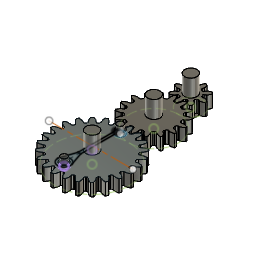
SqueezeFan v3 (Autodesk Fusion 360 design; units mm, degrees)
description: Spur Gear; Diametrial Pitch: 8.000000; Num Teeth: 24; Pressure Angle: 20.000000; Backlash: 0.00 in
description: Spur Gear; Diametrial Pitch: 8.000000; Num Teeth: 16; Pressure Angle: 20.000000; Backlash: 0.05 in
description: Spur Gear; Diametrial Pitch: 8.000000; Num Teeth: 8; Pressure Angle: 20.000000; Backlash: 0.00 in
Autodesk Fusion 360 part; units mm, degrees
(part 1 of 11)
sketch "Sketch1" plane through (0, 0, 0) normal (0, 0, 1) x (1, 0, 0) in component "Spur Gear (24 teeth)"
  circle A0 centre (0, 0) radius 34.2392
  circle A1 centre (0, 0) radius 6.35
extrude "Extrude1" add sketch "Sketch1" along normal blind 12.7 makes body 1 in component "Spur Gear (24 teeth)"
sketch "Sketch2" plane through (0, 0, 0) normal (0, 0, 1) x (1, 0, 0) in component "Spur Gear (24 teeth)"
  spline S0 degree 5 poles (35.6868, -2.8738) (35.7028, -2.8751) (35.735, -2.8772) (35.7832, -2.8793) (35.8475, -2.8797) (35.9281, -2.8771) (36.0087, -2.8722) (36.0893, -2.8659) (36.17, -2.8589) (36.2507, -2.8513) (36.3314, -2.8432) (36.4121, -2.8344) (36.4928, -2.8246) (36.5735, -2.8138) (36.6542, -2.8018) (36.7349, -2.7889) (36.8156, -2.775) (36.8963, -2.7604) (36.9769, -2.7452) (37.0576, -2.7294) (37.1382, -2.713) (37.2187, -2.696) (37.2993, -2.6783) (37.3798, -2.6599) (37.4603, -2.6409) (37.5408, -2.6212) (37.6212, -2.6008) (37.7016, -2.5799) (37.7819, -2.5584) (37.8622, -2.5364) (37.9425, -2.5139) (38.0227, -2.4907) (38.1029, -2.4671) (38.183, -2.4429) (38.2631, -2.4181) (38.3431, -2.3929) (38.4231, -2.3671) (38.503, -2.3408) (38.5829, -2.314) (38.6627, -2.2867) (38.7425, -2.2589) (38.8222, -2.2307) (38.9018, -2.2019) (38.9814, -2.1727) (39.061, -2.143) (39.1404, -2.1129) (39.2198, -2.0822) (39.2992, -2.0512) (39.3785, -2.0196) (39.4577, -1.9876) (39.5369, -1.9552) (39.6159, -1.9224) (39.695, -1.889) (39.7739, -1.8553) (39.8528, -1.8211) (39.9316, -1.7865) (40.0103, -1.7515) (40.089, -1.7161) (40.1676, -1.6802) (40.2461, -1.644) (40.3245, -1.6073) (40.4029, -1.5702) (40.4811, -1.5327) (40.5593, -1.4948) (40.6374, -1.4565) (40.7155, -1.4178) (40.7934, -1.3787) (40.8713, -1.3392) (40.9491, -1.2993) (41.0268, -1.259) (41.1044, -1.2184) (41.1664, -1.1855) (41.2129, -1.1607) (41.2439, -1.1441) (41.2594, -1.1358) knots 0 0 0 0 0 0 0.01428571 0.02857143 0.04285714 0.05714286 0.07142857 0.08571429 0.1 0.11428571 0.12857143 0.14285714 0.15714286 0.17142857 0.18571429 0.2 0.21428571 0.22857143 0.24285714 0.25714286 0.27142857 0.28571429 0.3 0.31428571 0.32857143 0.34285714 0.35714286 0.37142857 0.38571429 0.4 0.41428571 0.42857143 0.44285714 0.45714286 0.47142857 0.48571429 0.5 0.51428571 0.52857143 0.54285714 0.55714286 0.57142857 0.58571429 0.6 0.61428571 0.62857143 0.64285714 0.65714286 0.67142857 0.68571429 0.7 0.71428571 0.72857143 0.74285714 0.75714286 0.77142857 0.78571429 0.8 0.81428571 0.82857143 0.84285714 0.85714286 0.87142857 0.88571429 0.9 0.91428571 0.92857143 0.94285714 0.95714286 0.97142857 0.98571429 1 1 1 1 1 1
  spline S1 degree 5 poles (35.6868, 2.8738) (35.7028, 2.8751) (35.735, 2.8772) (35.7832, 2.8793) (35.8475, 2.8797) (35.9281, 2.8771) (36.0087, 2.8722) (36.0893, 2.8659) (36.17, 2.8589) (36.2507, 2.8513) (36.3314, 2.8432) (36.4121, 2.8344) (36.4928, 2.8246) (36.5735, 2.8138) (36.6542, 2.8018) (36.7349, 2.7889) (36.8156, 2.775) (36.8963, 2.7604) (36.9769, 2.7452) (37.0576, 2.7294) (37.1382, 2.713) (37.2187, 2.696) (37.2993, 2.6783) (37.3798, 2.6599) (37.4603, 2.6409) (37.5408, 2.6212) (37.6212, 2.6008) (37.7016, 2.5799) (37.7819, 2.5584) (37.8622, 2.5364) (37.9425, 2.5139) (38.0227, 2.4907) (38.1029, 2.4671) (38.183, 2.4429) (38.2631, 2.4181) (38.3431, 2.3929) (38.4231, 2.3671) (38.503, 2.3408) (38.5829, 2.314) (38.6627, 2.2867) (38.7425, 2.2589) (38.8222, 2.2307) (38.9018, 2.2019) (38.9814, 2.1727) (39.061, 2.143) (39.1404, 2.1129) (39.2198, 2.0822) (39.2992, 2.0512) (39.3785, 2.0196) (39.4577, 1.9876) (39.5369, 1.9552) (39.6159, 1.9224) (39.695, 1.889) (39.7739, 1.8553) (39.8528, 1.8211) (39.9316, 1.7865) (40.0103, 1.7515) (40.089, 1.7161) (40.1676, 1.6802) (40.2461, 1.644) (40.3245, 1.6073) (40.4029, 1.5702) (40.4811, 1.5327) (40.5593, 1.4948) (40.6374, 1.4565) (40.7155, 1.4178) (40.7934, 1.3787) (40.8713, 1.3392) (40.9491, 1.2993) (41.0268, 1.259) (41.1044, 1.2184) (41.1664, 1.1855) (41.2129, 1.1607) (41.2439, 1.1441) (41.2594, 1.1358) knots 0 0 0 0 0 0 0.01428571 0.02857143 0.04285714 0.05714286 0.07142857 0.08571429 0.1 0.11428571 0.12857143 0.14285714 0.15714286 0.17142857 0.18571429 0.2 0.21428571 0.22857143 0.24285714 0.25714286 0.27142857 0.28571429 0.3 0.31428571 0.32857143 0.34285714 0.35714286 0.37142857 0.38571429 0.4 0.41428571 0.42857143 0.44285714 0.45714286 0.47142857 0.48571429 0.5 0.51428571 0.52857143 0.54285714 0.55714286 0.57142857 0.58571429 0.6 0.61428571 0.62857143 0.64285714 0.65714286 0.67142857 0.68571429 0.7 0.71428571 0.72857143 0.74285714 0.75714286 0.77142857 0.78571429 0.8 0.81428571 0.82857143 0.84285714 0.85714286 0.87142857 0.88571429 0.9 0.91428571 0.92857143 0.94285714 0.95714286 0.97142857 0.98571429 1 1 1 1 1 1
  arc A0 (41.2594, -1.1358) -> (41.2594, 1.1358) centre (0, 0) ccw
  line L0 (34.1188, -2.7483) -> (35.6868, -2.8738)
  line L1 (34.1188, 2.7483) -> (35.6868, 2.8738)
  line L2 (34.1188, -2.7483) -> (34.1188, 2.7483)
  point P0 (36.0795, -2.8665)
  point P1 (36.4747, -2.8266)
  point P2 (36.8715, -2.7648)
  point P3 (37.2693, -2.6848)
  point P4 (37.668, -2.5886)
  point P5 (38.0672, -2.4775)
  point P6 (38.4668, -2.3526)
  point P7 (38.8665, -2.2146)
  point P8 (39.2663, -2.064)
  point P9 (39.6658, -1.9013)
  point P10 (40.0651, -1.7268)
  point P11 (40.4639, -1.5409)
  point P12 (40.862, -1.3438)
  point P13 (36.0795, 2.8665)
  point P14 (36.4747, 2.8266)
  point P15 (36.8715, 2.7648)
  point P16 (37.2693, 2.6848)
  point P17 (37.668, 2.5886)
  point P18 (38.0672, 2.4775)
  point P19 (38.4668, 2.3526)
  point P20 (38.8665, 2.2146)
  point P21 (39.2663, 2.064)
  point P22 (39.6658, 1.9013)
  point P23 (40.0651, 1.7268)
  point P24 (40.4639, 1.5409)
  point P25 (40.862, 1.3438)
extrude "Extrude2" add sketch "Sketch2" along normal blind 12.7 bodies 1 in component "Spur Gear (24 teeth)"
fillet "Fillet1" radius 1.5875 2 edges at (34.1287, -2.7491, 6.35) (34.1287, 2.7491, 6.35) on bodies 1 in component "Spur Gear (24 teeth)"
pattern_circular "C-Pattern1" count 24 over 360 about axis through (0, 0, 0) along (0, 0, 1) of "Extrude2", "Fillet1" in component "Spur Gear (24 teeth)"
sketch "Sketch3" plane through (0, 0, 0) normal (0, 0, 1) x (1, 0, 0) in component "Spur Gear (24 teeth)"
  circle A0 centre (0, 0) radius 38.1 construction
sketch "Sketch1 (2)" plane through (0, 0, 0) normal (0, 0, 1) x (1, 0, 0) in component "Spur Gear (16 teeth)"
  circle A0 centre (0, 0) radius 21.5392
  circle A1 centre (0, 0) radius 6.35
extrude "Extrude1'" add sketch "Sketch1 (2)" along normal blind 12.7 separate body makes body 2 in component "Spur Gear (16 teeth)"
sketch "Sketch2 (2)" plane through (0, 0, 0) normal (0, 0, 1) x (1, 0, 0) in component "Spur Gear (16 teeth)"
  spline S0 degree 5 poles (23.7476, -2.3966) (23.7615, -2.398) (23.7892, -2.4004) (23.831, -2.4028) (23.8867, -2.4037) (23.9564, -2.4017) (24.0263, -2.3975) (24.0962, -2.392) (24.1662, -2.3856) (24.2362, -2.3788) (24.3062, -2.3714) (24.3763, -2.3633) (24.4463, -2.3543) (24.5164, -2.3441) (24.5864, -2.3329) (24.6565, -2.3207) (24.7266, -2.3076) (24.7966, -2.2937) (24.8666, -2.2793) (24.9366, -2.2642) (25.0066, -2.2485) (25.0766, -2.2322) (25.1465, -2.2153) (25.2164, -2.1976) (25.2863, -2.1792) (25.3561, -2.1602) (25.4259, -2.1406) (25.4957, -2.1204) (25.5654, -2.0997) (25.6351, -2.0783) (25.7047, -2.0564) (25.7743, -2.034) (25.8439, -2.011) (25.9134, -1.9875) (25.9828, -1.9634) (26.0522, -1.9388) (26.1215, -1.9136) (26.1908, -1.888) (26.26, -1.8618) (26.3291, -1.8352) (26.3982, -1.808) (26.4672, -1.7803) (26.5362, -1.7522) (26.605, -1.7236) (26.6739, -1.6944) (26.7426, -1.6649) (26.8113, -1.6348) (26.8799, -1.6043) (26.9484, -1.5733) (27.0168, -1.5418) (27.0852, -1.5099) (27.1535, -1.4776) (27.2217, -1.4448) (27.2898, -1.4115) (27.3578, -1.3779) (27.4258, -1.3437) (27.4936, -1.3092) (27.5614, -1.2742) (27.6291, -1.2388) (27.6967, -1.2029) (27.7642, -1.1667) (27.8316, -1.13) (27.8989, -1.0929) (27.9661, -1.0554) (28.0332, -1.0175) (28.1002, -0.9792) (28.1671, -0.9404) (28.2339, -0.9013) (28.3007, -0.8618) (28.3673, -0.8218) (28.4338, -0.7815) (28.4869, -0.7489) (28.5267, -0.7243) (28.5532, -0.7078) (28.5664, -0.6995) knots 0 0 0 0 0 0 0.01428571 0.02857143 0.04285714 0.05714286 0.07142857 0.08571429 0.1 0.11428571 0.12857143 0.14285714 0.15714286 0.17142857 0.18571429 0.2 0.21428571 0.22857143 0.24285714 0.25714286 0.27142857 0.28571429 0.3 0.31428571 0.32857143 0.34285714 0.35714286 0.37142857 0.38571429 0.4 0.41428571 0.42857143 0.44285714 0.45714286 0.47142857 0.48571429 0.5 0.51428571 0.52857143 0.54285714 0.55714286 0.57142857 0.58571429 0.6 0.61428571 0.62857143 0.64285714 0.65714286 0.67142857 0.68571429 0.7 0.71428571 0.72857143 0.74285714 0.75714286 0.77142857 0.78571429 0.8 0.81428571 0.82857143 0.84285714 0.85714286 0.87142857 0.88571429 0.9 0.91428571 0.92857143 0.94285714 0.95714286 0.97142857 0.98571429 1 1 1 1 1 1
  spline S1 degree 5 poles (23.7476, 2.3966) (23.7615, 2.398) (23.7892, 2.4004) (23.831, 2.4028) (23.8867, 2.4037) (23.9564, 2.4017) (24.0263, 2.3975) (24.0962, 2.392) (24.1662, 2.3856) (24.2362, 2.3788) (24.3062, 2.3714) (24.3763, 2.3633) (24.4463, 2.3543) (24.5164, 2.3441) (24.5864, 2.3329) (24.6565, 2.3207) (24.7266, 2.3076) (24.7966, 2.2937) (24.8666, 2.2793) (24.9366, 2.2642) (25.0066, 2.2485) (25.0766, 2.2322) (25.1465, 2.2153) (25.2164, 2.1976) (25.2863, 2.1792) (25.3561, 2.1602) (25.4259, 2.1406) (25.4957, 2.1204) (25.5654, 2.0997) (25.6351, 2.0783) (25.7047, 2.0564) (25.7743, 2.034) (25.8439, 2.011) (25.9134, 1.9875) (25.9828, 1.9634) (26.0522, 1.9388) (26.1215, 1.9136) (26.1908, 1.888) (26.26, 1.8618) (26.3291, 1.8352) (26.3982, 1.808) (26.4672, 1.7803) (26.5362, 1.7522) (26.605, 1.7236) (26.6739, 1.6944) (26.7426, 1.6649) (26.8113, 1.6348) (26.8799, 1.6043) (26.9484, 1.5733) (27.0168, 1.5418) (27.0852, 1.5099) (27.1535, 1.4776) (27.2217, 1.4448) (27.2898, 1.4115) (27.3578, 1.3779) (27.4258, 1.3437) (27.4936, 1.3092) (27.5614, 1.2742) (27.6291, 1.2388) (27.6967, 1.2029) (27.7642, 1.1667) (27.8316, 1.13) (27.8989, 1.0929) (27.9661, 1.0554) (28.0332, 1.0175) (28.1002, 0.9792) (28.1671, 0.9404) (28.2339, 0.9013) (28.3007, 0.8618) (28.3673, 0.8218) (28.4338, 0.7815) (28.4869, 0.7489) (28.5267, 0.7243) (28.5532, 0.7078) (28.5664, 0.6995) knots 0 0 0 0 0 0 0.01428571 0.02857143 0.04285714 0.05714286 0.07142857 0.08571429 0.1 0.11428571 0.12857143 0.14285714 0.15714286 0.17142857 0.18571429 0.2 0.21428571 0.22857143 0.24285714 0.25714286 0.27142857 0.28571429 0.3 0.31428571 0.32857143 0.34285714 0.35714286 0.37142857 0.38571429 0.4 0.41428571 0.42857143 0.44285714 0.45714286 0.47142857 0.48571429 0.5 0.51428571 0.52857143 0.54285714 0.55714286 0.57142857 0.58571429 0.6 0.61428571 0.62857143 0.64285714 0.65714286 0.67142857 0.68571429 0.7 0.71428571 0.72857143 0.74285714 0.75714286 0.77142857 0.78571429 0.8 0.81428571 0.82857143 0.84285714 0.85714286 0.87142857 0.88571429 0.9 0.91428571 0.92857143 0.94285714 0.95714286 0.97142857 0.98571429 1 1 1 1 1 1
  arc A0 (28.5664, -0.6995) -> (28.5664, 0.6995) centre (0, 0) ccw
  line L0 (21.4204, -2.1627) -> (23.7476, -2.3966)
  line L1 (21.4204, 2.1627) -> (23.7476, 2.3966)
  line L2 (21.4204, -2.1627) -> (21.4204, 2.1627)
  point P0 (24.0858, -2.3926)
  point P1 (24.4272, -2.3566)
  point P2 (24.7704, -2.2988)
  point P3 (25.1148, -2.2229)
  point P4 (25.4602, -2.1306)
  point P5 (25.8062, -2.0234)
  point P6 (26.1525, -1.9021)
  point P7 (26.4989, -1.7673)
  point P8 (26.8452, -1.6196)
  point P9 (27.1911, -1.4594)
  point P10 (27.5363, -1.2871)
  point P11 (27.8808, -1.1028)
  point P12 (28.2242, -0.9069)
  point P13 (24.0858, 2.3926)
  point P14 (24.4272, 2.3566)
  point P15 (24.7704, 2.2988)
  point P16 (25.1148, 2.2229)
  point P17 (25.4602, 2.1306)
  point P18 (25.8062, 2.0234)
  point P19 (26.1525, 1.9021)
  point P20 (26.4989, 1.7673)
  point P21 (26.8452, 1.6196)
  point P22 (27.1911, 1.4594)
  point P23 (27.5363, 1.2871)
  point P24 (27.8808, 1.1028)
  point P25 (28.2242, 0.9069)
extrude "Extrude2'" add sketch "Sketch2 (2)" along normal blind 12.7 bodies 2 in component "Spur Gear (16 teeth)"
fillet "Fillet1'" radius 1.5875 2 edges at (21.4302, -2.1637, 6.35) (21.4302, 2.1637, 6.35) on bodies 2 in component "Spur Gear (16 teeth)"
pattern_circular "C-Pattern1'" count 16 over 360 about axis through (0, 0, 0) along (0, 0, 1) of "Extrude2'", "Fillet1'" in component "Spur Gear (16 teeth)"
sketch "Sketch3 (2)" plane through (0, 0, 0) normal (0, 0, 1) x (1, 0, 0) in component "Spur Gear (16 teeth)"
  circle A0 centre (0, 0) radius 25.4 construction
sketch "Sketch2 (3)" plane through (0, 0, 12.7) normal (0, 0, 1) x (-1, 0, 0)
  arc A0 (-33.9178, 4.6802) -> (-33.9734, 4.2579) centre (0, 0) ccw
  arc A1 (-35.6752, 2.8728) -> (-33.9734, 4.2579) centre (-35.5486, 4.4553) ccw
  line L0 (-35.6752, 2.8728) -> (-35.6868, 2.8738)
  spline S0 degree 5 poles (-35.6868, 2.8738) (-35.7028, 2.8751) (-35.735, 2.8772) (-35.7832, 2.8793) (-35.8475, 2.8797) (-35.9281, 2.8771) (-36.0087, 2.8722) (-36.0893, 2.8659) (-36.17, 2.8589) (-36.2507, 2.8513) (-36.3314, 2.8432) (-36.4121, 2.8344) (-36.4928, 2.8246) (-36.5735, 2.8138) (-36.6542, 2.8018) (-36.7349, 2.7889) (-36.8156, 2.775) (-36.8963, 2.7604) (-36.9769, 2.7452) (-37.0576, 2.7294) (-37.1382, 2.713) (-37.2187, 2.696) (-37.2993, 2.6783) (-37.3798, 2.6599) (-37.4603, 2.6409) (-37.5408, 2.6212) (-37.6212, 2.6008) (-37.7016, 2.5799) (-37.7819, 2.5584) (-37.8622, 2.5364) (-37.9425, 2.5139) (-38.0227, 2.4907) (-38.1029, 2.4671) (-38.183, 2.4429) (-38.2631, 2.4181) (-38.3431, 2.3929) (-38.4231, 2.3671) (-38.503, 2.3408) (-38.5829, 2.314) (-38.6627, 2.2867) (-38.7425, 2.2589) (-38.8222, 2.2307) (-38.9018, 2.2019) (-38.9814, 2.1727) (-39.061, 2.143) (-39.1404, 2.1129) (-39.2198, 2.0822) (-39.2992, 2.0512) (-39.3785, 2.0196) (-39.4577, 1.9876) (-39.5369, 1.9552) (-39.6159, 1.9224) (-39.695, 1.889) (-39.7739, 1.8553) (-39.8528, 1.8211) (-39.9316, 1.7865) (-40.0103, 1.7515) (-40.089, 1.7161) (-40.1676, 1.6802) (-40.2461, 1.644) (-40.3245, 1.6073) (-40.4029, 1.5702) (-40.4811, 1.5327) (-40.5593, 1.4948) (-40.6374, 1.4565) (-40.7155, 1.4178) (-40.7934, 1.3787) (-40.8713, 1.3392) (-40.9491, 1.2993) (-41.0268, 1.259) (-41.1044, 1.2184) (-41.1664, 1.1855) (-41.2129, 1.1607) (-41.2439, 1.1441) (-41.2594, 1.1358) knots 0 0 0 0 0 0 0.01428571 0.02857143 0.04285714 0.05714286 0.07142857 0.08571429 0.1 0.11428571 0.12857143 0.14285714 0.15714286 0.17142857 0.18571429 0.2 0.21428571 0.22857143 0.24285714 0.25714286 0.27142857 0.28571429 0.3 0.31428571 0.32857143 0.34285714 0.35714286 0.37142857 0.38571429 0.4 0.41428571 0.42857143 0.44285714 0.45714286 0.47142857 0.48571429 0.5 0.51428571 0.52857143 0.54285714 0.55714286 0.57142857 0.58571429 0.6 0.61428571 0.62857143 0.64285714 0.65714286 0.67142857 0.68571429 0.7 0.71428571 0.72857143 0.74285714 0.75714286 0.77142857 0.78571429 0.8 0.81428571 0.82857143 0.84285714 0.85714286 0.87142857 0.88571429 0.9 0.91428571 0.92857143 0.94285714 0.95714286 0.97142857 0.98571429 1 1 1 1 1 1
  arc A2 (-41.2594, 1.1358) -> (-41.2594, -1.1358) centre (0, 0) ccw
  spline S1 degree 5 poles (-41.2594, -1.1358) (-41.2439, -1.1441) (-41.2129, -1.1607) (-41.1664, -1.1855) (-41.1044, -1.2184) (-41.0268, -1.259) (-40.9491, -1.2993) (-40.8713, -1.3392) (-40.7934, -1.3787) (-40.7155, -1.4178) (-40.6374, -1.4565) (-40.5593, -1.4948) (-40.4811, -1.5327) (-40.4029, -1.5702) (-40.3245, -1.6073) (-40.2461, -1.644) (-40.1676, -1.6802) (-40.089, -1.7161) (-40.0103, -1.7515) (-39.9316, -1.7865) (-39.8528, -1.8211) (-39.7739, -1.8553) (-39.695, -1.889) (-39.6159, -1.9224) (-39.5369, -1.9552) (-39.4577, -1.9876) (-39.3785, -2.0196) (-39.2992, -2.0512) (-39.2198, -2.0822) (-39.1404, -2.1129) (-39.061, -2.143) (-38.9814, -2.1727) (-38.9018, -2.2019) (-38.8222, -2.2307) (-38.7425, -2.2589) (-38.6627, -2.2867) (-38.5829, -2.314) (-38.503, -2.3408) (-38.4231, -2.3671) (-38.3431, -2.3929) (-38.2631, -2.4181) (-38.183, -2.4429) (-38.1029, -2.4671) (-38.0227, -2.4907) (-37.9425, -2.5139) (-37.8622, -2.5364) (-37.7819, -2.5584) (-37.7016, -2.5799) (-37.6212, -2.6008) (-37.5408, -2.6212) (-37.4603, -2.6409) (-37.3798, -2.6599) (-37.2993, -2.6783) (-37.2187, -2.696) (-37.1382, -2.713) (-37.0576, -2.7294) (-36.9769, -2.7452) (-36.8963, -2.7604) (-36.8156, -2.775) (-36.7349, -2.7889) (-36.6542, -2.8018) (-36.5735, -2.8138) (-36.4928, -2.8246) (-36.4121, -2.8344) (-36.3314, -2.8432) (-36.2507, -2.8513) (-36.17, -2.8589) (-36.0893, -2.8659) (-36.0087, -2.8722) (-35.9281, -2.8771) (-35.8475, -2.8797) (-35.7832, -2.8793) (-35.735, -2.8772) (-35.7028, -2.8751) (-35.6868, -2.8738) knots -1 -1 -1 -1 -1 -1 -0.98571429 -0.97142857 -0.95714286 -0.94285714 -0.92857143 -0.91428571 -0.9 -0.88571429 -0.87142857 -0.85714286 -0.84285714 -0.82857143 -0.81428571 -0.8 -0.78571429 -0.77142857 -0.75714286 -0.74285714 -0.72857143 -0.71428571 -0.7 -0.68571429 -0.67142857 -0.65714286 -0.64285714 -0.62857143 -0.61428571 -0.6 -0.58571429 -0.57142857 -0.55714286 -0.54285714 -0.52857143 -0.51428571 -0.5 -0.48571429 -0.47142857 -0.45714286 -0.44285714 -0.42857143 -0.41428571 -0.4 -0.38571429 -0.37142857 -0.35714286 -0.34285714 -0.32857143 -0.31428571 -0.3 -0.28571429 -0.27142857 -0.25714286 -0.24285714 -0.22857143 -0.21428571 -0.2 -0.18571429 -0.17142857 -0.15714286 -0.14285714 -0.12857143 -0.11428571 -0.1 -0.08571429 -0.07142857 -0.05714286 -0.04285714 -0.02857143 -0.01428571 0 0 0 0 0 0
  line L1 (-35.6868, -2.8738) -> (-35.6752, -2.8728)
  arc A3 (-33.9734, -4.2579) -> (-35.6752, -2.8728) centre (-35.5486, -4.4553) ccw
  arc A4 (-33.9734, -4.2579) -> (-33.9178, -4.6802) centre (0, 0) ccw
  arc A5 (-35.2032, -6.4585) -> (-33.9178, -4.6802) centre (-35.4904, -4.8972) ccw
  line L2 (-35.2032, -6.4585) -> (-35.2146, -6.4606)
  spline S2 degree 5 poles (-35.2146, -6.4606) (-35.2304, -6.4635) (-35.262, -6.4697) (-35.3091, -6.4802) (-35.3714, -6.4965) (-35.4485, -6.5198) (-35.5251, -6.5454) (-35.6014, -6.5723) (-35.6775, -6.6) (-35.7535, -6.6282) (-35.8293, -6.6569) (-35.905, -6.6863) (-35.9804, -6.7167) (-36.0556, -6.748) (-36.1304, -6.7805) (-36.205, -6.8139) (-36.2794, -6.8481) (-36.3535, -6.8831) (-36.4275, -6.9186) (-36.5013, -6.9548) (-36.5749, -6.9915) (-36.6483, -7.0288) (-36.7215, -7.0667) (-36.7946, -7.1053) (-36.8674, -7.1446) (-36.94, -7.1844) (-37.0124, -7.2249) (-37.0846, -7.2659) (-37.1567, -7.3074) (-37.2286, -7.3495) (-37.3002, -7.392) (-37.3717, -7.4351) (-37.4431, -7.4787) (-37.5142, -7.5228) (-37.5851, -7.5675) (-37.6559, -7.6126) (-37.7265, -7.6582) (-37.7969, -7.7043) (-37.8671, -7.7508) (-37.9371, -7.7979) (-38.007, -7.8453) (-38.0767, -7.8933) (-38.1462, -7.9416) (-38.2155, -7.9905) (-38.2846, -8.0397) (-38.3536, -8.0894) (-38.4224, -8.1396) (-38.491, -8.1901) (-38.5594, -8.2411) (-38.6277, -8.2925) (-38.6957, -8.3443) (-38.7636, -8.3965) (-38.8313, -8.4491) (-38.8988, -8.5022) (-38.9662, -8.5556) (-39.0333, -8.6094) (-39.1003, -8.6636) (-39.1671, -8.7182) (-39.2338, -8.7732) (-39.3002, -8.8285) (-39.3665, -8.8842) (-39.4326, -8.9404) (-39.4985, -8.9968) (-39.5642, -9.0537) (-39.6297, -9.1109) (-39.6951, -9.1685) (-39.7603, -9.2264) (-39.8253, -9.2847) (-39.8901, -9.3434) (-39.9547, -9.4024) (-40.0191, -9.4618) (-40.0706, -9.5095) (-40.109, -9.5455) (-40.1347, -9.5696) (-40.1475, -9.5816) knots 0 0 0 0 0 0 0.01428571 0.02857143 0.04285714 0.05714286 0.07142857 0.08571429 0.1 0.11428571 0.12857143 0.14285714 0.15714286 0.17142857 0.18571429 0.2 0.21428571 0.22857143 0.24285714 0.25714286 0.27142857 0.28571429 0.3 0.31428571 0.32857143 0.34285714 0.35714286 0.37142857 0.38571429 0.4 0.41428571 0.42857143 0.44285714 0.45714286 0.47142857 0.48571429 0.5 0.51428571 0.52857143 0.54285714 0.55714286 0.57142857 0.58571429 0.6 0.61428571 0.62857143 0.64285714 0.65714286 0.67142857 0.68571429 0.7 0.71428571 0.72857143 0.74285714 0.75714286 0.77142857 0.78571429 0.8 0.81428571 0.82857143 0.84285714 0.85714286 0.87142857 0.88571429 0.9 0.91428571 0.92857143 0.94285714 0.95714286 0.97142857 0.98571429 1 1 1 1 1 1
  arc A6 (-40.1475, -9.5816) -> (-39.5595, -11.7758) centre (0, 0) ccw
  spline S3 degree 5 poles (-39.5595, -11.7758) (-39.5424, -11.7798) (-39.5082, -11.7879) (-39.4569, -11.7998) (-39.3885, -11.8154) (-39.303, -11.8346) (-39.2175, -11.8534) (-39.132, -11.8718) (-39.0466, -11.8898) (-38.9612, -11.9074) (-38.8758, -11.9246) (-38.7904, -11.9414) (-38.7051, -11.9577) (-38.6198, -11.9737) (-38.5345, -11.9892) (-38.4492, -12.0044) (-38.364, -12.0191) (-38.2788, -12.0334) (-38.1937, -12.0473) (-38.1086, -12.0607) (-38.0235, -12.0737) (-37.9384, -12.0863) (-37.8535, -12.0985) (-37.7685, -12.1102) (-37.6836, -12.1215) (-37.5988, -12.1323) (-37.514, -12.1427) (-37.4292, -12.1526) (-37.3445, -12.1621) (-37.2599, -12.1711) (-37.1753, -12.1797) (-37.0908, -12.1878) (-37.0064, -12.1954) (-36.922, -12.2026) (-36.8377, -12.2092) (-36.7535, -12.2154) (-36.6693, -12.2211) (-36.5852, -12.2263) (-36.5012, -12.231) (-36.4173, -12.2353) (-36.3334, -12.239) (-36.2497, -12.2421) (-36.166, -12.2448) (-36.0824, -12.2469) (-35.999, -12.2484) (-35.9156, -12.2495) (-35.8323, -12.2499) (-35.7492, -12.2499) (-35.6661, -12.2493) (-35.5832, -12.2481) (-35.5004, -12.2463) (-35.4177, -12.2439) (-35.3352, -12.2408) (-35.2528, -12.2371) (-35.1705, -12.2327) (-35.0884, -12.2276) (-35.0065, -12.222) (-34.9246, -12.2159) (-34.8429, -12.2091) (-34.7614, -12.2015) (-34.6801, -12.1932) (-34.5991, -12.1838) (-34.5183, -12.1734) (-34.4378, -12.162) (-34.3576, -12.1496) (-34.2775, -12.1365) (-34.1976, -12.1229) (-34.1179, -12.1089) (-34.0383, -12.0941) (-33.9592, -12.0779) (-33.8808, -12.0596) (-33.8187, -12.0425) (-33.7726, -12.0281) (-33.7422, -12.0177) (-33.727, -12.0123) knots -1 -1 -1 -1 -1 -1 -0.98571429 -0.97142857 -0.95714286 -0.94285714 -0.92857143 -0.91428571 -0.9 -0.88571429 -0.87142857 -0.85714286 -0.84285714 -0.82857143 -0.81428571 -0.8 -0.78571429 -0.77142857 -0.75714286 -0.74285714 -0.72857143 -0.71428571 -0.7 -0.68571429 -0.67142857 -0.65714286 -0.64285714 -0.62857143 -0.61428571 -0.6 -0.58571429 -0.57142857 -0.55714286 -0.54285714 -0.52857143 -0.51428571 -0.5 -0.48571429 -0.47142857 -0.45714286 -0.44285714 -0.42857143 -0.41428571 -0.4 -0.38571429 -0.37142857 -0.35714286 -0.34285714 -0.32857143 -0.31428571 -0.3 -0.28571429 -0.27142857 -0.25714286 -0.24285714 -0.22857143 -0.21428571 -0.2 -0.18571429 -0.17142857 -0.15714286 -0.14285714 -0.12857143 -0.11428571 -0.1 -0.08571429 -0.07142857 -0.05714286 -0.04285714 -0.02857143 -0.01428571 0 0 0 0 0 0
  line L3 (-33.727, -12.0123) -> (-33.7161, -12.0084)
  arc A7 (-31.7138, -12.9058) -> (-33.7161, -12.0084) centre (-33.1842, -13.5041) ccw
  arc A8 (-31.7138, -12.9058) -> (-31.5508, -13.2993) centre (0, 0) ccw
  arc A9 (-32.3321, -15.3497) -> (-31.5508, -13.2993) centre (-33.0136, -13.9159) ccw
  line L4 (-32.3321, -15.3497) -> (-32.3425, -15.3546)
  spline S4 degree 5 poles (-32.3425, -15.3546) (-32.3571, -15.3615) (-32.386, -15.3757) (-32.4288, -15.3981) (-32.4847, -15.4299) (-32.5532, -15.4724) (-32.6205, -15.5169) (-32.6872, -15.5627) (-32.7536, -15.6091) (-32.8197, -15.656) (-32.8855, -15.7034) (-32.951, -15.7514) (-33.016, -15.8002) (-33.0805, -15.85) (-33.1444, -15.9007) (-33.2078, -15.9522) (-33.2708, -16.0046) (-33.3333, -16.0575) (-33.3956, -16.111) (-33.4575, -16.165) (-33.5191, -16.2195) (-33.5804, -16.2746) (-33.6413, -16.3302) (-33.7018, -16.3863) (-33.762, -16.4431) (-33.8218, -16.5004) (-33.8813, -16.5582) (-33.9405, -16.6165) (-33.9993, -16.6753) (-34.0578, -16.7345) (-34.1161, -16.7942) (-34.174, -16.8543) (-34.2316, -16.9149) (-34.2889, -16.9759) (-34.3459, -17.0374) (-34.4025, -17.0993) (-34.4589, -17.1616) (-34.515, -17.2243) (-34.5707, -17.2875) (-34.6262, -17.351) (-34.6814, -17.4149) (-34.7363, -17.4793) (-34.7909, -17.544) (-34.8453, -17.6091) (-34.8993, -17.6746) (-34.953, -17.7404) (-35.0065, -17.8067) (-35.0597, -17.8733) (-35.1126, -17.9402) (-35.1652, -18.0075) (-35.2175, -18.0752) (-35.2696, -18.1432) (-35.3214, -18.2115) (-35.3729, -18.2802) (-35.4241, -18.3492) (-35.475, -18.4186) (-35.5257, -18.4883) (-35.5761, -18.5583) (-35.6262, -18.6287) (-35.6761, -18.6993) (-35.7257, -18.7703) (-35.775, -18.8416) (-35.824, -18.9132) (-35.8728, -18.9852) (-35.9213, -19.0574) (-35.9695, -19.1299) (-36.0175, -19.2028) (-36.0652, -19.2759) (-36.1126, -19.3493) (-36.1598, -19.4231) (-36.2066, -19.4971) (-36.2439, -19.5565) (-36.2718, -19.6012) (-36.2903, -19.6311) (-36.2996, -19.6461) knots 0 0 0 0 0 0 0.01428571 0.02857143 0.04285714 0.05714286 0.07142857 0.08571429 0.1 0.11428571 0.12857143 0.14285714 0.15714286 0.17142857 0.18571429 0.2 0.21428571 0.22857143 0.24285714 0.25714286 0.27142857 0.28571429 0.3 0.31428571 0.32857143 0.34285714 0.35714286 0.37142857 0.38571429 0.4 0.41428571 0.42857143 0.44285714 0.45714286 0.47142857 0.48571429 0.5 0.51428571 0.52857143 0.54285714 0.55714286 0.57142857 0.58571429 0.6 0.61428571 0.62857143 0.64285714 0.65714286 0.67142857 0.68571429 0.7 0.71428571 0.72857143 0.74285714 0.75714286 0.77142857 0.78571429 0.8 0.81428571 0.82857143 0.84285714 0.85714286 0.87142857 0.88571429 0.9 0.91428571 0.92857143 0.94285714 0.95714286 0.97142857 0.98571429 1 1 1 1 1 1
  arc A10 (-36.2996, -19.6461) -> (-35.1638, -21.6133) centre (0, 0) ccw
  spline S5 degree 5 poles (-35.1638, -21.6133) (-35.1462, -21.6128) (-35.1111, -21.6117) (-35.0584, -21.6099) (-34.9883, -21.6073) (-34.9007, -21.6037) (-34.8133, -21.5998) (-34.726, -21.5954) (-34.6388, -21.5907) (-34.5518, -21.5856) (-34.4648, -21.5801) (-34.378, -21.5742) (-34.2914, -21.5679) (-34.2048, -21.5612) (-34.1184, -21.5542) (-34.0321, -21.5467) (-33.946, -21.5389) (-33.86, -21.5307) (-33.7742, -21.522) (-33.6885, -21.513) (-33.6029, -21.5035) (-33.5176, -21.4937) (-33.4323, -21.4834) (-33.3472, -21.4728) (-33.2623, -21.4617) (-33.1776, -21.4502) (-33.093, -21.4383) (-33.0085, -21.4259) (-32.9243, -21.4132) (-32.8402, -21.4) (-32.7563, -21.3864) (-32.6726, -21.3723) (-32.589, -21.3578) (-32.5057, -21.3429) (-32.4225, -21.3275) (-32.3395, -21.3117) (-32.2568, -21.2954) (-32.1742, -21.2787) (-32.0918, -21.2615) (-32.0097, -21.2438) (-31.9277, -21.2257) (-31.846, -21.2071) (-31.7645, -21.188) (-31.6832, -21.1684) (-31.6022, -21.1483) (-31.5214, -21.1277) (-31.4409, -21.1066) (-31.3605, -21.0851) (-31.2805, -21.063) (-31.2007, -21.0404) (-31.1211, -21.0172) (-31.0419, -20.9935) (-30.963, -20.9691) (-30.8844, -20.9442) (-30.8061, -20.9186) (-30.7281, -20.8925) (-30.6503, -20.8659) (-30.5729, -20.8388) (-30.4957, -20.8111) (-30.419, -20.7827) (-30.3426, -20.7536) (-30.2667, -20.7236) (-30.1914, -20.6926) (-30.1166, -20.6607) (-30.0423, -20.628) (-29.9684, -20.5947) (-29.8947, -20.5609) (-29.8213, -20.5266) (-29.7483, -20.4917) (-29.6761, -20.4557) (-29.605, -20.4177) (-29.5495, -20.3851) (-29.5088, -20.3592) (-29.482, -20.3413) (-29.4688, -20.3321) knots -1 -1 -1 -1 -1 -1 -0.98571429 -0.97142857 -0.95714286 -0.94285714 -0.92857143 -0.91428571 -0.9 -0.88571429 -0.87142857 -0.85714286 -0.84285714 -0.82857143 -0.81428571 -0.8 -0.78571429 -0.77142857 -0.75714286 -0.74285714 -0.72857143 -0.71428571 -0.7 -0.68571429 -0.67142857 -0.65714286 -0.64285714 -0.62857143 -0.61428571 -0.6 -0.58571429 -0.57142857 -0.55714286 -0.54285714 -0.52857143 -0.51428571 -0.5 -0.48571429 -0.47142857 -0.45714286 -0.44285714 -0.42857143 -0.41428571 -0.4 -0.38571429 -0.37142857 -0.35714286 -0.34285714 -0.32857143 -0.31428571 -0.3 -0.28571429 -0.27142857 -0.25714286 -0.24285714 -0.22857143 -0.21428571 -0.2 -0.18571429 -0.17142857 -0.15714286 -0.14285714 -0.12857143 -0.11428571 -0.1 -0.08571429 -0.07142857 -0.05714286 -0.04285714 -0.02857143 -0.01428571 0 0 0 0 0 0
  line L5 (-29.4688, -20.3321) -> (-29.4592, -20.3256)
  arc A11 (-27.2929, -20.6741) -> (-29.4592, -20.3256) centre (-28.5583, -21.6327) ccw
  arc A12 (-27.2929, -20.6741) -> (-27.0336, -21.0121) centre (0, 0) ccw
  arc A13 (-27.2576, -23.1948) -> (-27.0336, -21.0121) centre (-28.287, -21.9863) ccw
  line L6 (-27.2576, -23.1948) -> (-27.2664, -23.2023)
  spline S6 degree 5 poles (-27.2664, -23.2023) (-27.2787, -23.2127) (-27.3029, -23.2339) (-27.3385, -23.2666) (-27.3843, -23.3118) (-27.4394, -23.3706) (-27.4929, -23.431) (-27.5455, -23.4925) (-27.5976, -23.5545) (-27.6493, -23.6169) (-27.7006, -23.6797) (-27.7515, -23.743) (-27.8016, -23.807) (-27.851, -23.8718) (-27.8997, -23.9373) (-27.9475, -24.0035) (-27.9948, -24.0703) (-28.0415, -24.1377) (-28.0878, -24.2055) (-28.1337, -24.2736) (-28.1791, -24.3422) (-28.224, -24.4113) (-28.2684, -24.4807) (-28.3124, -24.5507) (-28.3558, -24.6211) (-28.3988, -24.6919) (-28.4413, -24.7631) (-28.4833, -24.8347) (-28.5249, -24.9067) (-28.5661, -24.9791) (-28.6069, -25.0518) (-28.6473, -25.1249) (-28.6873, -25.1983) (-28.7268, -25.2721) (-28.766, -25.3462) (-28.8047, -25.4206) (-28.843, -25.4954) (-28.8809, -25.5705) (-28.9185, -25.646) (-28.9556, -25.7217) (-28.9924, -25.7978) (-29.0287, -25.8741) (-29.0647, -25.9508) (-29.1004, -26.0277) (-29.1356, -26.1049) (-29.1705, -26.1825) (-29.205, -26.2603) (-29.2391, -26.3383) (-29.2729, -26.4167) (-29.3063, -26.4953) (-29.3393, -26.5742) (-29.372, -26.6534) (-29.4043, -26.7328) (-29.4363, -26.8125) (-29.4679, -26.8924) (-29.4992, -26.9726) (-29.5301, -27.053) (-29.5606, -27.1337) (-29.5909, -27.2147) (-29.6207, -27.2958) (-29.6502, -27.3772) (-29.6794, -27.4589) (-29.7082, -27.5407) (-29.7367, -27.6228) (-29.7649, -27.7051) (-29.7927, -27.7877) (-29.8202, -27.8705) (-29.8473, -27.9534) (-29.8741, -28.0366) (-29.9006, -28.1201) (-29.9267, -28.2037) (-29.9474, -28.2708) (-29.9627, -28.3212) (-29.9728, -28.3548) (-29.9779, -28.3717) knots 0 0 0 0 0 0 0.01428571 0.02857143 0.04285714 0.05714286 0.07142857 0.08571429 0.1 0.11428571 0.12857143 0.14285714 0.15714286 0.17142857 0.18571429 0.2 0.21428571 0.22857143 0.24285714 0.25714286 0.27142857 0.28571429 0.3 0.31428571 0.32857143 0.34285714 0.35714286 0.37142857 0.38571429 0.4 0.41428571 0.42857143 0.44285714 0.45714286 0.47142857 0.48571429 0.5 0.51428571 0.52857143 0.54285714 0.55714286 0.57142857 0.58571429 0.6 0.61428571 0.62857143 0.64285714 0.65714286 0.67142857 0.68571429 0.7 0.71428571 0.72857143 0.74285714 0.75714286 0.77142857 0.78571429 0.8 0.81428571 0.82857143 0.84285714 0.85714286 0.87142857 0.88571429 0.9 0.91428571 0.92857143 0.94285714 0.95714286 0.97142857 0.98571429 1 1 1 1 1 1
  arc A14 (-29.9779, -28.3717) -> (-28.3717, -29.9779) centre (0, 0) ccw
  spline S7 degree 5 poles (-28.3717, -29.9779) (-28.3548, -29.9728) (-28.3212, -29.9627) (-28.2708, -29.9474) (-28.2037, -29.9267) (-28.1201, -29.9006) (-28.0366, -29.8741) (-27.9534, -29.8473) (-27.8705, -29.8202) (-27.7877, -29.7927) (-27.7051, -29.7649) (-27.6228, -29.7367) (-27.5407, -29.7082) (-27.4589, -29.6794) (-27.3772, -29.6502) (-27.2958, -29.6207) (-27.2147, -29.5909) (-27.1337, -29.5606) (-27.053, -29.5301) (-26.9726, -29.4992) (-26.8924, -29.4679) (-26.8125, -29.4363) (-26.7328, -29.4043) (-26.6534, -29.372) (-26.5742, -29.3393) (-26.4953, -29.3063) (-26.4167, -29.2729) (-26.3383, -29.2391) (-26.2603, -29.205) (-26.1825, -29.1705) (-26.1049, -29.1356) (-26.0277, -29.1004) (-25.9508, -29.0647) (-25.8741, -29.0287) (-25.7978, -28.9924) (-25.7217, -28.9556) (-25.646, -28.9185) (-25.5705, -28.8809) (-25.4954, -28.843) (-25.4206, -28.8047) (-25.3462, -28.766) (-25.2721, -28.7268) (-25.1983, -28.6873) (-25.1249, -28.6473) (-25.0518, -28.6069) (-24.9791, -28.5661) (-24.9067, -28.5249) (-24.8347, -28.4833) (-24.7631, -28.4413) (-24.6919, -28.3988) (-24.6211, -28.3558) (-24.5507, -28.3124) (-24.4807, -28.2684) (-24.4113, -28.224) (-24.3422, -28.1791) (-24.2736, -28.1337) (-24.2055, -28.0878) (-24.1377, -28.0415) (-24.0703, -27.9948) (-24.0035, -27.9475) (-23.9373, -27.8997) (-23.8718, -27.851) (-23.807, -27.8016) (-23.743, -27.7515) (-23.6797, -27.7006) (-23.6169, -27.6493) (-23.5545, -27.5976) (-23.4925, -27.5455) (-23.431, -27.4929) (-23.3706, -27.4394) (-23.3118, -27.3843) (-23.2666, -27.3385) (-23.2339, -27.3029) (-23.2127, -27.2787) (-23.2023, -27.2664) knots -1 -1 -1 -1 -1 -1 -0.98571429 -0.97142857 -0.95714286 -0.94285714 -0.92857143 -0.91428571 -0.9 -0.88571429 -0.87142857 -0.85714286 -0.84285714 -0.82857143 -0.81428571 -0.8 -0.78571429 -0.77142857 -0.75714286 -0.74285714 -0.72857143 -0.71428571 -0.7 -0.68571429 -0.67142857 -0.65714286 -0.64285714 -0.62857143 -0.61428571 -0.6 -0.58571429 -0.57142857 -0.55714286 -0.54285714 -0.52857143 -0.51428571 -0.5 -0.48571429 -0.47142857 -0.45714286 -0.44285714 -0.42857143 -0.41428571 -0.4 -0.38571429 -0.37142857 -0.35714286 -0.34285714 -0.32857143 -0.31428571 -0.3 -0.28571429 -0.27142857 -0.25714286 -0.24285714 -0.22857143 -0.21428571 -0.2 -0.18571429 -0.17142857 -0.15714286 -0.14285714 -0.12857143 -0.11428571 -0.1 -0.08571429 -0.07142857 -0.05714286 -0.04285714 -0.02857143 -0.01428571 0 0 0 0 0 0
  line L7 (-23.2023, -27.2664) -> (-23.1948, -27.2576)
  arc A15 (-21.0121, -27.0336) -> (-23.1948, -27.2576) centre (-21.9863, -28.287) ccw
  arc A16 (-21.0121, -27.0336) -> (-20.6741, -27.2929) centre (0, 0) ccw
  arc A17 (-20.3256, -29.4592) -> (-20.6741, -27.2929) centre (-21.6327, -28.5583) ccw
  line L8 (-20.3256, -29.4592) -> (-20.3321, -29.4688)
  spline S8 degree 5 poles (-20.3321, -29.4688) (-20.3413, -29.482) (-20.3592, -29.5088) (-20.3851, -29.5495) (-20.4177, -29.605) (-20.4557, -29.6761) (-20.4917, -29.7483) (-20.5266, -29.8213) (-20.5609, -29.8947) (-20.5947, -29.9684) (-20.628, -30.0423) (-20.6607, -30.1166) (-20.6926, -30.1914) (-20.7236, -30.2667) (-20.7536, -30.3426) (-20.7827, -30.419) (-20.8111, -30.4957) (-20.8388, -30.5729) (-20.8659, -30.6503) (-20.8925, -30.7281) (-20.9186, -30.8061) (-20.9442, -30.8844) (-20.9691, -30.963) (-20.9935, -31.0419) (-21.0172, -31.1211) (-21.0404, -31.2007) (-21.063, -31.2805) (-21.0851, -31.3605) (-21.1066, -31.4409) (-21.1277, -31.5214) (-21.1483, -31.6022) (-21.1684, -31.6832) (-21.188, -31.7645) (-21.2071, -31.846) (-21.2257, -31.9277) (-21.2438, -32.0097) (-21.2615, -32.0918) (-21.2787, -32.1742) (-21.2954, -32.2568) (-21.3117, -32.3395) (-21.3275, -32.4225) (-21.3429, -32.5057) (-21.3578, -32.589) (-21.3723, -32.6726) (-21.3864, -32.7563) (-21.4, -32.8402) (-21.4132, -32.9243) (-21.4259, -33.0085) (-21.4383, -33.093) (-21.4502, -33.1776) (-21.4617, -33.2623) (-21.4728, -33.3472) (-21.4834, -33.4323) (-21.4937, -33.5176) (-21.5035, -33.6029) (-21.513, -33.6885) (-21.522, -33.7742) (-21.5307, -33.86) (-21.5389, -33.946) (-21.5467, -34.0321) (-21.5542, -34.1184) (-21.5612, -34.2048) (-21.5679, -34.2914) (-21.5742, -34.378) (-21.5801, -34.4648) (-21.5856, -34.5518) (-21.5907, -34.6388) (-21.5954, -34.726) (-21.5998, -34.8133) (-21.6037, -34.9007) (-21.6073, -34.9883) (-21.6099, -35.0584) (-21.6117, -35.1111) (-21.6128, -35.1462) (-21.6133, -35.1638) knots 0 0 0 0 0 0 0.01428571 0.02857143 0.04285714 0.05714286 0.07142857 0.08571429 0.1 0.11428571 0.12857143 0.14285714 0.15714286 0.17142857 0.18571429 0.2 0.21428571 0.22857143 0.24285714 0.25714286 0.27142857 0.28571429 0.3 0.31428571 0.32857143 0.34285714 0.35714286 0.37142857 0.38571429 0.4 0.41428571 0.42857143 0.44285714 0.45714286 0.47142857 0.48571429 0.5 0.51428571 0.52857143 0.54285714 0.55714286 0.57142857 0.58571429 0.6 0.61428571 0.62857143 0.64285714 0.65714286 0.67142857 0.68571429 0.7 0.71428571 0.72857143 0.74285714 0.75714286 0.77142857 0.78571429 0.8 0.81428571 0.82857143 0.84285714 0.85714286 0.87142857 0.88571429 0.9 0.91428571 0.92857143 0.94285714 0.95714286 0.97142857 0.98571429 1 1 1 1 1 1
  arc A18 (-21.6133, -35.1638) -> (-19.6461, -36.2996) centre (0, 0) ccw
  spline S9 degree 5 poles (-19.6461, -36.2996) (-19.6311, -36.2903) (-19.6012, -36.2718) (-19.5565, -36.2439) (-19.4971, -36.2066) (-19.4231, -36.1598) (-19.3493, -36.1126) (-19.2759, -36.0652) (-19.2028, -36.0175) (-19.1299, -35.9695) (-19.0574, -35.9213) (-18.9852, -35.8728) (-18.9132, -35.824) (-18.8416, -35.775) (-18.7703, -35.7257) (-18.6993, -35.6761) (-18.6287, -35.6262) (-18.5583, -35.5761) (-18.4883, -35.5257) (-18.4186, -35.475) (-18.3492, -35.4241) (-18.2802, -35.3729) (-18.2115, -35.3214) (-18.1432, -35.2696) (-18.0752, -35.2175) (-18.0075, -35.1652) (-17.9402, -35.1126) (-17.8733, -35.0597) (-17.8067, -35.0065) (-17.7404, -34.953) (-17.6746, -34.8993) (-17.6091, -34.8453) (-17.544, -34.7909) (-17.4793, -34.7363) (-17.4149, -34.6814) (-17.351, -34.6262) (-17.2875, -34.5707) (-17.2243, -34.515) (-17.1616, -34.4589) (-17.0993, -34.4025) (-17.0374, -34.3459) (-16.9759, -34.2889) (-16.9149, -34.2316) (-16.8543, -34.174) (-16.7942, -34.1161) (-16.7345, -34.0578) (-16.6753, -33.9993) (-16.6165, -33.9405) (-16.5582, -33.8813) (-16.5004, -33.8218) (-16.4431, -33.762) (-16.3863, -33.7018) (-16.3302, -33.6413) (-16.2746, -33.5804) (-16.2195, -33.5191) (-16.165, -33.4575) (-16.111, -33.3956) (-16.0575, -33.3333) (-16.0046, -33.2708) (-15.9522, -33.2078) (-15.9007, -33.1444) (-15.85, -33.0805) (-15.8002, -33.016) (-15.7514, -32.951) (-15.7034, -32.8855) (-15.656, -32.8197) (-15.6091, -32.7536) (-15.5627, -32.6872) (-15.5169, -32.6205) (-15.4724, -32.5532) (-15.4299, -32.4847) (-15.3981, -32.4288) (-15.3757, -32.386) (-15.3615, -32.3571) (-15.3546, -32.3425) knots -1 -1 -1 -1 -1 -1 -0.98571429 -0.97142857 -0.95714286 -0.94285714 -0.92857143 -0.91428571 -0.9 -0.88571429 -0.87142857 -0.85714286 -0.84285714 -0.82857143 -0.81428571 -0.8 -0.78571429 -0.77142857 -0.75714286 -0.74285714 -0.72857143 -0.71428571 -0.7 -0.68571429 -0.67142857 -0.65714286 -0.64285714 -0.62857143 -0.61428571 -0.6 -0.58571429 -0.57142857 -0.55714286 -0.54285714 -0.52857143 -0.51428571 -0.5 -0.48571429 -0.47142857 -0.45714286 -0.44285714 -0.42857143 -0.41428571 -0.4 -0.38571429 -0.37142857 -0.35714286 -0.34285714 -0.32857143 -0.31428571 -0.3 -0.28571429 -0.27142857 -0.25714286 -0.24285714 -0.22857143 -0.21428571 -0.2 -0.18571429 -0.17142857 -0.15714286 -0.14285714 -0.12857143 -0.11428571 -0.1 -0.08571429 -0.07142857 -0.05714286 -0.04285714 -0.02857143 -0.01428571 0 0 0 0 0 0
  line L9 (-15.3546, -32.3425) -> (-15.3497, -32.3321)
  arc A19 (-13.2993, -31.5508) -> (-15.3497, -32.3321) centre (-13.9159, -33.0136) ccw
  arc A20 (-13.2993, -31.5508) -> (-12.9058, -31.7138) centre (0, 0) ccw
  arc A21 (-12.0084, -33.7161) -> (-12.9058, -31.7138) centre (-13.5041, -33.1842) ccw
  line L10 (-12.0084, -33.7161) -> (-12.0123, -33.727)
  spline S10 degree 5 poles (-12.0123, -33.727) (-12.0177, -33.7422) (-12.0281, -33.7726) (-12.0425, -33.8187) (-12.0596, -33.8808) (-12.0779, -33.9592) (-12.0941, -34.0383) (-12.1089, -34.1179) (-12.1229, -34.1976) (-12.1365, -34.2775) (-12.1496, -34.3576) (-12.162, -34.4378) (-12.1734, -34.5183) (-12.1838, -34.5991) (-12.1932, -34.6801) (-12.2015, -34.7614) (-12.2091, -34.8429) (-12.2159, -34.9246) (-12.222, -35.0065) (-12.2276, -35.0884) (-12.2327, -35.1705) (-12.2371, -35.2528) (-12.2408, -35.3352) (-12.2439, -35.4177) (-12.2463, -35.5004) (-12.2481, -35.5832) (-12.2493, -35.6661) (-12.2499, -35.7492) (-12.2499, -35.8323) (-12.2495, -35.9156) (-12.2484, -35.999) (-12.2469, -36.0824) (-12.2448, -36.166) (-12.2421, -36.2497) (-12.239, -36.3334) (-12.2353, -36.4173) (-12.231, -36.5012) (-12.2263, -36.5852) (-12.2211, -36.6693) (-12.2154, -36.7535) (-12.2092, -36.8377) (-12.2026, -36.922) (-12.1954, -37.0064) (-12.1878, -37.0908) (-12.1797, -37.1753) (-12.1711, -37.2599) (-12.1621, -37.3445) (-12.1526, -37.4292) (-12.1427, -37.514) (-12.1323, -37.5988) (-12.1215, -37.6836) (-12.1102, -37.7685) (-12.0985, -37.8535) (-12.0863, -37.9384) (-12.0737, -38.0235) (-12.0607, -38.1086) (-12.0473, -38.1937) (-12.0334, -38.2788) (-12.0191, -38.364) (-12.0044, -38.4492) (-11.9892, -38.5345) (-11.9737, -38.6198) (-11.9577, -38.7051) (-11.9414, -38.7904) (-11.9246, -38.8758) (-11.9074, -38.9612) (-11.8898, -39.0466) (-11.8718, -39.132) (-11.8534, -39.2175) (-11.8346, -39.303) (-11.8154, -39.3885) (-11.7998, -39.4569) (-11.7879, -39.5082) (-11.7798, -39.5424) (-11.7758, -39.5595) knots 0 0 0 0 0 0 0.01428571 0.02857143 0.04285714 0.05714286 0.07142857 0.08571429 0.1 0.11428571 0.12857143 0.14285714 0.15714286 0.17142857 0.18571429 0.2 0.21428571 0.22857143 0.24285714 0.25714286 0.27142857 0.28571429 0.3 0.31428571 0.32857143 0.34285714 0.35714286 0.37142857 0.38571429 0.4 0.41428571 0.42857143 0.44285714 0.45714286 0.47142857 0.48571429 0.5 0.51428571 0.52857143 0.54285714 0.55714286 0.57142857 0.58571429 0.6 0.61428571 0.62857143 0.64285714 0.65714286 0.67142857 0.68571429 0.7 0.71428571 0.72857143 0.74285714 0.75714286 0.77142857 0.78571429 0.8 0.81428571 0.82857143 0.84285714 0.85714286 0.87142857 0.88571429 0.9 0.91428571 0.92857143 0.94285714 0.95714286 0.97142857 0.98571429 1 1 1 1 1 1
  arc A22 (-11.7758, -39.5595) -> (-9.5816, -40.1475) centre (0, 0) ccw
  spline S11 degree 5 poles (-9.5816, -40.1475) (-9.5696, -40.1347) (-9.5455, -40.109) (-9.5095, -40.0706) (-9.4618, -40.0191) (-9.4024, -39.9547) (-9.3434, -39.8901) (-9.2847, -39.8253) (-9.2264, -39.7603) (-9.1685, -39.6951) (-9.1109, -39.6297) (-9.0537, -39.5642) (-8.9968, -39.4985) (-8.9404, -39.4326) (-8.8842, -39.3665) (-8.8285, -39.3002) (-8.7732, -39.2338) (-8.7182, -39.1671) (-8.6636, -39.1003) (-8.6094, -39.0333) (-8.5556, -38.9662) (-8.5022, -38.8988) (-8.4491, -38.8313) (-8.3965, -38.7636) (-8.3443, -38.6957) (-8.2925, -38.6277) (-8.2411, -38.5594) (-8.1901, -38.491) (-8.1396, -38.4224) (-8.0894, -38.3536) (-8.0397, -38.2846) (-7.9905, -38.2155) (-7.9416, -38.1462) (-7.8933, -38.0767) (-7.8453, -38.007) (-7.7979, -37.9371) (-7.7508, -37.8671) (-7.7043, -37.7969) (-7.6582, -37.7265) (-7.6126, -37.6559) (-7.5675, -37.5851) (-7.5228, -37.5142) (-7.4787, -37.4431) (-7.4351, -37.3717) (-7.392, -37.3002) (-7.3495, -37.2286) (-7.3074, -37.1567) (-7.2659, -37.0846) (-7.2249, -37.0124) (-7.1844, -36.94) (-7.1446, -36.8674) (-7.1053, -36.7946) (-7.0667, -36.7215) (-7.0288, -36.6483) (-6.9915, -36.5749) (-6.9548, -36.5013) (-6.9186, -36.4275) (-6.8831, -36.3535) (-6.8481, -36.2794) (-6.8139, -36.205) (-6.7805, -36.1304) (-6.748, -36.0556) (-6.7167, -35.9804) (-6.6863, -35.905) (-6.6569, -35.8293) (-6.6282, -35.7535) (-6.6, -35.6775) (-6.5723, -35.6014) (-6.5454, -35.5251) (-6.5198, -35.4485) (-6.4965, -35.3714) (-6.4802, -35.3091) (-6.4697, -35.262) (-6.4635, -35.2304) (-6.4606, -35.2146) knots -1 -1 -1 -1 -1 -1 -0.98571429 -0.97142857 -0.95714286 -0.94285714 -0.92857143 -0.91428571 -0.9 -0.88571429 -0.87142857 -0.85714286 -0.84285714 -0.82857143 -0.81428571 -0.8 -0.78571429 -0.77142857 -0.75714286 -0.74285714 -0.72857143 -0.71428571 -0.7 -0.68571429 -0.67142857 -0.65714286 -0.64285714 -0.62857143 -0.61428571 -0.6 -0.58571429 -0.57142857 -0.55714286 -0.54285714 -0.52857143 -0.51428571 -0.5 -0.48571429 -0.47142857 -0.45714286 -0.44285714 -0.42857143 -0.41428571 -0.4 -0.38571429 -0.37142857 -0.35714286 -0.34285714 -0.32857143 -0.31428571 -0.3 -0.28571429 -0.27142857 -0.25714286 -0.24285714 -0.22857143 -0.21428571 -0.2 -0.18571429 -0.17142857 -0.15714286 -0.14285714 -0.12857143 -0.11428571 -0.1 -0.08571429 -0.07142857 -0.05714286 -0.04285714 -0.02857143 -0.01428571 0 0 0 0 0 0
  line L11 (-6.4606, -35.2146) -> (-6.4585, -35.2032)
  arc A23 (-4.6802, -33.9178) -> (-6.4585, -35.2032) centre (-4.8972, -35.4904) ccw
  arc A24 (-4.6802, -33.9178) -> (-4.2579, -33.9734) centre (0, 0) ccw
  arc A25 (-2.8728, -35.6752) -> (-4.2579, -33.9734) centre (-4.4553, -35.5486) ccw
  line L12 (-2.8728, -35.6752) -> (-2.8738, -35.6868)
  spline S12 degree 5 poles (-2.8738, -35.6868) (-2.8751, -35.7028) (-2.8772, -35.735) (-2.8793, -35.7832) (-2.8797, -35.8475) (-2.8771, -35.9281) (-2.8722, -36.0087) (-2.8659, -36.0893) (-2.8589, -36.17) (-2.8513, -36.2507) (-2.8432, -36.3314) (-2.8344, -36.4121) (-2.8246, -36.4928) (-2.8138, -36.5735) (-2.8018, -36.6542) (-2.7889, -36.7349) (-2.775, -36.8156) (-2.7604, -36.8963) (-2.7452, -36.9769) (-2.7294, -37.0576) (-2.713, -37.1382) (-2.696, -37.2187) (-2.6783, -37.2993) (-2.6599, -37.3798) (-2.6409, -37.4603) (-2.6212, -37.5408) (-2.6008, -37.6212) (-2.5799, -37.7016) (-2.5584, -37.7819) (-2.5364, -37.8622) (-2.5139, -37.9425) (-2.4907, -38.0227) (-2.4671, -38.1029) (-2.4429, -38.183) (-2.4181, -38.2631) (-2.3929, -38.3431) (-2.3671, -38.4231) (-2.3408, -38.503) (-2.314, -38.5829) (-2.2867, -38.6627) (-2.2589, -38.7425) (-2.2307, -38.8222) (-2.2019, -38.9018) (-2.1727, -38.9814) (-2.143, -39.061) (-2.1129, -39.1404) (-2.0822, -39.2198) (-2.0512, -39.2992) (-2.0196, -39.3785) (-1.9876, -39.4577) (-1.9552, -39.5369) (-1.9224, -39.6159) (-1.889, -39.695) (-1.8553, -39.7739) (-1.8211, -39.8528) (-1.7865, -39.9316) (-1.7515, -40.0103) (-1.7161, -40.089) (-1.6802, -40.1676) (-1.644, -40.2461) (-1.6073, -40.3245) (-1.5702, -40.4029) (-1.5327, -40.4811) (-1.4948, -40.5593) (-1.4565, -40.6374) (-1.4178, -40.7155) (-1.3787, -40.7934) (-1.3392, -40.8713) (-1.2993, -40.9491) (-1.259, -41.0268) (-1.2184, -41.1044) (-1.1855, -41.1664) (-1.1607, -41.2129) (-1.1441, -41.2439) (-1.1358, -41.2594) knots 0 0 0 0 0 0 0.01428571 0.02857143 0.04285714 0.05714286 0.07142857 0.08571429 0.1 0.11428571 0.12857143 0.14285714 0.15714286 0.17142857 0.18571429 0.2 0.21428571 0.22857143 0.24285714 0.25714286 0.27142857 0.28571429 0.3 0.31428571 0.32857143 0.34285714 0.35714286 0.37142857 0.38571429 0.4 0.41428571 0.42857143 0.44285714 0.45714286 0.47142857 0.48571429 0.5 0.51428571 0.52857143 0.54285714 0.55714286 0.57142857 0.58571429 0.6 0.61428571 0.62857143 0.64285714 0.65714286 0.67142857 0.68571429 0.7 0.71428571 0.72857143 0.74285714 0.75714286 0.77142857 0.78571429 0.8 0.81428571 0.82857143 0.84285714 0.85714286 0.87142857 0.88571429 0.9 0.91428571 0.92857143 0.94285714 0.95714286 0.97142857 0.98571429 1 1 1 1 1 1
  arc A26 (-1.1358, -41.2594) -> (1.1358, -41.2594) centre (0, 0) ccw
  spline S13 degree 5 poles (1.1358, -41.2594) (1.1441, -41.2439) (1.1607, -41.2129) (1.1855, -41.1664) (1.2184, -41.1044) (1.259, -41.0268) (1.2993, -40.9491) (1.3392, -40.8713) (1.3787, -40.7934) (1.4178, -40.7155) (1.4565, -40.6374) (1.4948, -40.5593) (1.5327, -40.4811) (1.5702, -40.4029) (1.6073, -40.3245) (1.644, -40.2461) (1.6802, -40.1676) (1.7161, -40.089) (1.7515, -40.0103) (1.7865, -39.9316) (1.8211, -39.8528) (1.8553, -39.7739) (1.889, -39.695) (1.9224, -39.6159) (1.9552, -39.5369) (1.9876, -39.4577) (2.0196, -39.3785) (2.0512, -39.2992) (2.0822, -39.2198) (2.1129, -39.1404) (2.143, -39.061) (2.1727, -38.9814) (2.2019, -38.9018) (2.2307, -38.8222) (2.2589, -38.7425) (2.2867, -38.6627) (2.314, -38.5829) (2.3408, -38.503) (2.3671, -38.4231) (2.3929, -38.3431) (2.4181, -38.2631) (2.4429, -38.183) (2.4671, -38.1029) (2.4907, -38.0227) (2.5139, -37.9425) (2.5364, -37.8622) (2.5584, -37.7819) (2.5799, -37.7016) (2.6008, -37.6212) (2.6212, -37.5408) (2.6409, -37.4603) (2.6599, -37.3798) (2.6783, -37.2993) (2.696, -37.2187) (2.713, -37.1382) (2.7294, -37.0576) (2.7452, -36.9769) (2.7604, -36.8963) (2.775, -36.8156) (2.7889, -36.7349) (2.8018, -36.6542) (2.8138, -36.5735) (2.8246, -36.4928) (2.8344, -36.4121) (2.8432, -36.3314) (2.8513, -36.2507) (2.8589, -36.17) (2.8659, -36.0893) (2.8722, -36.0087) (2.8771, -35.9281) (2.8797, -35.8475) (2.8793, -35.7832) (2.8772, -35.735) (2.8751, -35.7028) (2.8738, -35.6868) knots -1 -1 -1 -1 -1 -1 -0.98571429 -0.97142857 -0.95714286 -0.94285714 -0.92857143 -0.91428571 -0.9 -0.88571429 -0.87142857 -0.85714286 -0.84285714 -0.82857143 -0.81428571 -0.8 -0.78571429 -0.77142857 -0.75714286 -0.74285714 -0.72857143 -0.71428571 -0.7 -0.68571429 -0.67142857 -0.65714286 -0.64285714 -0.62857143 -0.61428571 -0.6 -0.58571429 -0.57142857 -0.55714286 -0.54285714 -0.52857143 -0.51428571 -0.5 -0.48571429 -0.47142857 -0.45714286 -0.44285714 -0.42857143 -0.41428571 -0.4 -0.38571429 -0.37142857 -0.35714286 -0.34285714 -0.32857143 -0.31428571 -0.3 -0.28571429 -0.27142857 -0.25714286 -0.24285714 -0.22857143 -0.21428571 -0.2 -0.18571429 -0.17142857 -0.15714286 -0.14285714 -0.12857143 -0.11428571 -0.1 -0.08571429 -0.07142857 -0.05714286 -0.04285714 -0.02857143 -0.01428571 0 0 0 0 0 0
  line L13 (2.8738, -35.6868) -> (2.8728, -35.6752)
  arc A27 (4.2579, -33.9734) -> (2.8728, -35.6752) centre (4.4553, -35.5486) ccw
  arc A28 (4.2579, -33.9734) -> (4.6802, -33.9178) centre (0, 0) ccw
  arc A29 (6.4585, -35.2032) -> (4.6802, -33.9178) centre (4.8972, -35.4904) ccw
  line L14 (6.4585, -35.2032) -> (6.4606, -35.2146)